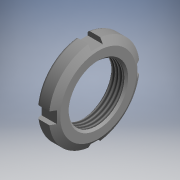
# Autodesk Inventor part: SKF_KM 5
Saved by Autodesk Inventor 2017.3 (Build 213256000, 256)
## iProperties
Part Number: SKF_KM 5
Material: Generic
Catalog Web Link: www.cadenas.de
Description: ANL_001-KM(L) and HM .. T lock nuts
Vendor: SKF
Document SubType Name: Modeling
Designer: partserver
Manufacturer: SKF
Mass: 28 g
Surface Area: 25.0949 cm^2
Volume: 4.31475 cm^3
Density: 1 g/cm^3
Appearance: PSOLRGB-175-175-175
Category: PARTsolutions
Company: SKF
Title: SKF_KM 5
Author: Cadenas PARTsolutions
Comments: KM(L) and HM .. T lock nuts
PSOL_IDENT_0: {$CADENAS_DATA\23d-libs\skf\bearings_units_and_housings\bearing_accessories\lock_nuts\anl_001.prj},1
PSOL_IDENT_1: 59 {VTYP=3D},{NB=SKF_KM 5},{LINA=SKF_KM 5},{NN=ANL_001},{DATE=13.09.2021 11:18:37},{GEOMDATE=10.09.2
PSOL_IDENT_2: 021 08:23:06},{VERSION=},{LINEID=3240},{WBVAR=},{WBNUMERIC=}  {NB=SKF_KM 5},{LINA=SKF_KM 5},{KT=DUMM
PSOL_IDENT_3: Y},{DESIGNATION=KM 5},{G=M 25x1.5},{DD=25.000},{TP=1.500},{DD3=38.000},{B=7.000},{DD1=32.000},{DD2=M
PSOL_IDENT_4: IN},{B3=MIN},{B5=MIN},{BB=5.000},{HH=2.000},{MASS=0.028},{SD=HN 5-6},{WD=MB 5},{DESIGN=locknut_km},{
PSOL_IDENT_5: LNB=34.000},{POPULAR=Yes},{LC=},{LCA=0},{LOAD=31.5},{WDX=MB 5},{KH=},{LCAA=0.000}
NB: SKF_KM 5
NN: ANL_001
NT: KM(L) and HM .. T lock nuts
NBSYN: SKF_$DESIGNATION.
LINA: SKF_KM 5
CATALOG: SKF
DESIGNATION: KM 5
G: M 25x1.5
DD: 25
DD3: 38
B: 7
WD: MB 5
POPULAR: Yes
LOAD: 31.5
WDX: MB 5
SUPPLIER: SKF
ARTICLENO: SKF_KM 5
BOMINFO: SKF_KM 5
CREATOR: CADENAS GmbH
Autodesk Inventor part; units mm, degrees
ref_plane "YZ Plane" through (0, 0, 0) normal (1, 0, 0) x (0, 1, 0)
ref_plane "XZ Plane" through (0, 0, 0) normal (0, 1, 0) x (-1, 0, 0)
ref_plane "XY Plane" through (0, 0, 0) normal (0, 0, 1) x (1, 0, 0)
sketch "Sketch_3" plane through (0, 0, 0) normal (0, 0, 1) x (1, 0, 0)
  line L0 (68, 0) -> (-68, 0)
  line L1 (0, 12.5) -> (0.812, 11.688)
  line L2 (0.812, 11.688) -> (6.188, 11.688)
  line L3 (6.188, 11.688) -> (7, 12.5)
  line L4 (7, 12.5) -> (7, 17.8333)
  arc A0 (7, 17.8333) -> (5.8333, 19) centre (5.8333, 17.8333) ccw
  line L5 (5.8333, 19) -> (1.7321, 19)
  line L6 (1.7321, 19) -> (0, 16)
  line L7 (0, 16) -> (0, 12.5)
  constraints: 16 end point, 2 point on circle, 1 centre point
revolve "Revolution1" add sketch "Sketch_3" angle 360 about axis through (68, 0, 0) along (-1, 0, 0)
thread "Thread1" size "M25x1.5" class "6H" standard "ISO Metric profile" full length
sketch "Sketch_6" plane through (0, 0, 0) normal (1, 0, 0) x (0, 1, 0)
  circle A0 centre (0, 0) radius 38
  line L0 (2.5, 23.8694) -> (2.5, 16.8348)
  line L1 (2.5, 16.8348) -> (-2.5, 16.8348)
  line L2 (-2.5, 16.8348) -> (-2.5, 23.8694)
  arc A1 (-2.5, 23.8694) -> (-23.8694, 2.5) centre (0, 0) ccw
  line L3 (-23.8694, 2.5) -> (-16.8348, 2.5)
  line L4 (-16.8348, 2.5) -> (-16.8348, -2.5)
  line L5 (-16.8348, -2.5) -> (-23.8694, -2.5)
  arc A2 (-23.8694, -2.5) -> (-2.5, -23.8694) centre (0, 0) ccw
  line L6 (-2.5, -23.8694) -> (-2.5, -16.8348)
  line L7 (-2.5, -16.8348) -> (2.5, -16.8348)
  line L8 (2.5, -16.8348) -> (2.5, -23.8694)
  arc A3 (2.5, -23.8694) -> (23.8694, -2.5) centre (0, 0) ccw
  line L9 (23.8694, -2.5) -> (16.8348, -2.5)
  line L10 (16.8348, -2.5) -> (16.8348, 2.5)
  line L11 (16.8348, 2.5) -> (23.8694, 2.5)
  arc A4 (23.8694, 2.5) -> (2.5, 23.8694) centre (0, 0) ccw
  constraints: 24 end point, 8 point on circle, 5 centre point
extrude "Extrusion1" cut sketch "Sketch_6" along normal blind 14
ref_plane "km_XY" through (7, 0, 0) normal (1, 0, 0) x (0, 0, -1)
ref_plane "km_YZ" through (7, 0, 0) normal (0, 0, -1) x (0, 1, 0)
ref_plane "km_ZX" through (7, 0, 0) normal (0, 1, 0) x (1, 0, 0)
ref_plane "km2_XY" through (7, 0, 0) normal (1, 0, 0) x (0, 0, -1)
ref_plane "km2_YZ" through (7, 0, 0) normal (0, 0, -1) x (0, 1, 0)
ref_plane "km2_ZX" through (7, 0, 0) normal (0, 1, 0) x (1, 0, 0)
ref_plane "ln_XY" through (0, 0, 0) normal (0, 1, 0) x (1, 0, 0)
ref_plane "ln_YZ" through (0, 0, 0) normal (1, 0, 0) x (0, 0, -1)
ref_plane "ln_ZX" through (0, 0, 0) normal (0, 0, -1) x (0, 1, 0)
ref_plane "nut_XY" through (0, 0, 0) normal (1, 0, 0) x (0, 0, -1)
ref_plane "nut_YZ" through (0, 0, 0) normal (0, 0, -1) x (0, 1, 0)
ref_plane "nut_ZX" through (0, 0, 0) normal (0, 1, 0) x (1, 0, 0)
body "Solid1"
